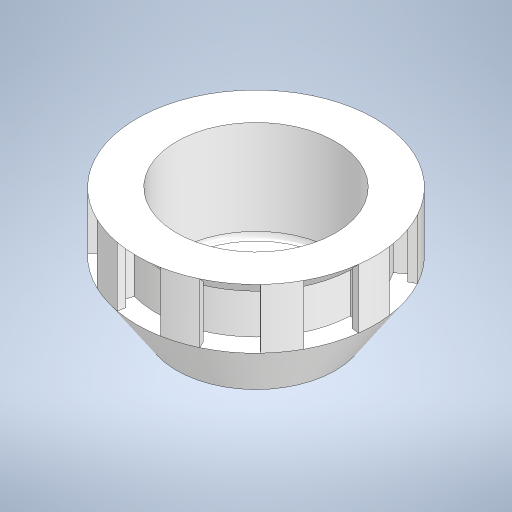
# Autodesk Inventor part: Tire Hub
Saved by Autodesk Inventor 2023.2 (Build 272271000, 271)
## iProperties
Created: 2023-02-06
Part Number: Tire Hub
Material: Nylon 6/6
Document SubType Name: Modeling
Designer: Nathan Cai
Density: 1.13 g/cm^3
Appearance: Smooth - White
Mass: 9.60807 g
Surface Area: 58.4208 cm^2
Volume: 8.50272 cm^3
Author: Nathan Cai
Autodesk Inventor part; units mm, degrees
ref_plane "YZ Plane" through (0, 0, 0) normal (1, 0, 0) x (0, 1, 0)
ref_plane "XZ Plane" through (0, 0, 0) normal (0, 1, 0) x (-1, 0, 0)
ref_plane "XY Plane" through (0, 0, 0) normal (0, 0, 1) x (1, 0, 0)
sketch "Sketch1" plane through (0, 0, 0) normal (0, 0, 1) x (1, 0, 0)
  line L0 (0, 19.05) -> (15.875, 19.05)
  line L1 (0, 9.525) -> (15.875, 9.525)
  line L2 (15.875, 19.05) -> (15.875, 9.525)
  line L3 (0, 0) -> (0, 19.05)
  line L4 (0, 19.05) -> (12.7, 19.05)
  line L5 (0, 0) -> (12.7, 0)
  line L6 (12.7, 0) -> (12.7, 19.05)
  line L7 (12.7, 19.05) -> (0, 19.05)
  line L8 (0, 19.05) -> (0, 0)
  line L9 (12.7, 3.175) -> (0, 3.175)
  line L10 (14.2875, 19.05) -> (14.2875, 9.525)
  line L11 (12.7, 0) -> (15.875, 0)
  line L12 (15.875, 0) -> (15.875, 9.525)
  line L13 (15.875, 9.525) -> (12.7, 9.525)
  line L14 (12.7, 9.525) -> (12.7, 0)
  line L15 (15.875, 0) -> (19.05, 9.525)
  line L16 (19.05, 9.525) -> (15.875, 9.525)
  line L17 (19.05, 9.525) -> (12.7, 0)
  point P0 (0, 3.175)
  dimension "d2" = 15.875
  dimension "d3" = 9.525
  dimension "d5" = 12.7
  dimension "d6" = 19.05
  dimension "d7" = 3.175
  dimension "d8" = 1.5875
  dimension "d21" = 19.05
  constraints: 36 end point, 6 horizontal, 4 parallel, 4 perpendicular, 4 point on line, 2 vertical
  measures "d2" distance of L0.start L0.end
  measures "d3" distance between parallel lines of L1 L0
  measures "d5" distance of L7.end L4.end
  measures "d6" distance between parallel lines of L5 L0
  measures "d7" distance between parallel lines of L5 L9
  measures "d8" distance between parallel lines of L2 L10
  measures "d21" distance from line of L3 L15.end
revolve "Revolution1" add sketch "Sketch1" angle 360 about axis through (0, 0, 0) along (0, 1, 0) contours L0 L10 L1 L6 | L0 L2 L1 L10 | L1 L12 L17 L6 | L9 L6 L5 L3 | L16 L17 L12
sketch "Sketch2" plane through (0, 0, 0) normal (0, -1, 0) x (1, 0, 0)
  circle A0 centre (0, 0) radius 3.302
  line L0 (0, 0) -> (0, -7.9375) construction
  circle A1 centre (0, -7.9375) radius 1.7526
  circle A2 centre (0, 7.9375) radius 1.7526
  point P0 (0, 0)
  dimension "d10" = 6.604
  dimension "d11" = 7.9375
  dimension "d12" = 3.5052
  dimension "d15" = 360
  constraints: 3 centre point, 2 coincident, 2 end point, 1 vertical, 5 other
  measures "d10" diameter of A0
  measures "d11" distance of L0.start L0.end
  measures "d12" diameter of A1
extrude "Extrusion1" cut sketch "Sketch2" against normal blind 25.4
fillet "Fillet1" radius 0.7937 1 edges at (-12.7, 3.175, 0)
chamfer "Chamfer1" distance 1.7272 angle 59 2 edges at (-1.7526, 0, 7.9375) (-1.7526, 0, -7.9375) measured on face at (-2.2526, 0, -7.9375) measured on face at (-2.2526, 0, 7.9375)
sketch "Sketch5" plane through (0, 19.05, 0) normal (0, 1, 0) x (1, 0, 0)
  circle A0 centre (0, 0) radius 19.05
  circle A1 centre (0, 0) radius 15.875
  dimension "d41" = 38.1
  constraints: 2 centre point, 1 coincident, 2 other
  measures "d41" diameter of A0
extrude "Extrusion3" add sketch "Sketch5" against normal blind 3.175
chamfer "Chamfer3" distance 3.175 angle 45 1 edges at (-19.05, 15.875, 0)
sketch "Sketch3" plane through (0, 9.525, 0) normal (0, 1, 0) x (1, 0, 0)
  circle A0 centre (0, 0) radius 19.05
  circle A1 centre (0, 0) radius 15.875
  circle A2 centre (0, 0) radius 17.8594
  line L0 (0, 0) -> (-19.0335, 0)
  line L1 (-19.0335, 0) -> (-19.0335, 0.7937) construction
  line L2 (-19.0335, 0.7937) -> (0, 0.7937)
  line L3 (0, 0.7937) -> (0, 0)
  line L4 (-19.0335, -0.7937) -> (0, -0.7937)
  circle A3 centre (0, 0) radius 19.05 projected
  line L5 (-17.7066, 2.3311) -> (-18.887, 2.4865)
  line L6 (-17.7066, -2.3311) -> (-18.887, -2.4865)
  line L7 (-15.8649, -10.5454) -> (-0.4666, 0.6422)
  line L8 (-14.9318, -11.8297) -> (0.4666, -0.6422)
  line L9 (-12.9547, -12.2936) -> (-13.8184, -13.1132)
  line L10 (-15.6951, -8.5218) -> (-16.7415, -9.0899)
  line L11 (-6.6366, -17.8566) -> (-0.7549, 0.2453)
  line L12 (-5.1268, -18.3472) -> (0.7549, -0.2453)
  line L13 (-3.2546, -17.5603) -> (-3.4716, -18.731)
  line L14 (-7.6887, -16.1196) -> (-8.2012, -17.1942)
  line L15 (5.1268, -18.3472) -> (-0.7549, -0.2453)
  line L16 (6.6366, -17.8566) -> (0.7549, 0.2453)
  line L17 (7.6887, -16.1196) -> (8.2012, -17.1942)
  line L18 (3.2546, -17.5603) -> (3.4716, -18.731)
  line L19 (14.9318, -11.8297) -> (-0.4666, -0.6422)
  line L20 (15.8649, -10.5454) -> (0.4666, 0.6422)
  line L21 (15.6951, -8.5218) -> (16.7415, -9.0899)
  line L22 (12.9547, -12.2936) -> (13.8184, -13.1132)
  line L23 (19.0335, -0.7938) -> (0, -0.7937)
  line L24 (19.0335, 0.7937) -> (0, 0.7937)
  line L25 (17.7066, 2.3311) -> (18.887, 2.4865)
  line L26 (17.7066, -2.3311) -> (18.887, -2.4865)
  line L27 (15.8649, 10.5454) -> (0.4666, -0.6422)
  line L28 (14.9318, 11.8297) -> (-0.4666, 0.6422)
  line L29 (12.9547, 12.2936) -> (13.8184, 13.1132)
  line L30 (15.6951, 8.5218) -> (16.7415, 9.0899)
  line L31 (6.6366, 17.8566) -> (0.7549, -0.2453)
  line L32 (5.1268, 18.3472) -> (-0.7549, 0.2453)
  line L33 (3.2546, 17.5603) -> (3.4716, 18.731)
  line L34 (7.6887, 16.1196) -> (8.2012, 17.1942)
  line L35 (-5.1268, 18.3472) -> (0.7549, 0.2453)
  line L36 (-6.6366, 17.8566) -> (-0.7549, -0.2453)
  line L37 (-7.6887, 16.1196) -> (-8.2012, 17.1942)
  line L38 (-3.2546, 17.5603) -> (-3.4716, 18.731)
  line L39 (-14.9318, 11.8297) -> (0.4666, 0.6422)
  line L40 (-15.8649, 10.5454) -> (-0.4666, -0.6422)
  line L41 (-15.6951, 8.5218) -> (-16.7415, 9.0899)
  line L42 (-12.9547, 12.2936) -> (-13.8184, 13.1132)
  point P0 (-13.9677, -11.1293)
  point P1 (-12.3605, -9.9616)
  point P2 (-13.2936, -8.6773)
  point P3 (-14.9008, -9.8449)
  point P4 (-4.7585, -17.2138)
  point P5 (-4.1446, -15.3244)
  point P6 (-5.6544, -14.8339)
  point P7 (-6.2683, -16.7232)
  point P8 (6.2683, -16.7232)
  point P9 (5.6544, -14.8339)
  point P10 (4.1446, -15.3244)
  point P11 (4.7585, -17.2138)
  point P12 (14.9008, -9.8449)
  point P13 (13.2936, -8.6773)
  point P14 (12.3605, -9.9616)
  point P15 (13.9677, -11.1293)
  point P16 (17.8417, 0.7937)
  point P17 (15.8551, 0.7937)
  point P18 (15.8551, -0.7938)
  point P19 (17.8417, -0.7938)
  point P20 (13.9677, 11.1293)
  point P21 (12.3605, 9.9616)
  point P22 (13.2936, 8.6773)
  point P23 (14.9008, 9.8449)
  point P24 (4.7585, 17.2138)
  point P25 (4.1446, 15.3244)
  point P26 (5.6544, 14.8339)
  point P27 (6.2683, 16.7232)
  point P28 (-6.2683, 16.7232)
  point P29 (-5.6544, 14.8339)
  point P30 (-4.1446, 15.3244)
  point P31 (-4.7585, 17.2138)
  point P32 (-14.9008, 9.8449)
  point P33 (-13.2936, 8.6773)
  point P34 (-12.3605, 9.9616)
  point P35 (-13.9677, 11.1293)
  point P36 (-17.8417, -0.7938)
  point P37 (-15.8551, -0.7938)
  point P38 (-15.8551, 0.7937)
  point P39 (-17.8417, 0.7937)
  dimension "d25" = 38.1
  dimension "d27" = 1.1906
  dimension "d26" = 31.75
  dimension "d28" = 0.7937
  dimension "d30" = 7.5
  dimension "d33" = 360
  constraints: 86 end point, 10 point on line, 4 symmetric about line, 3 coincident, 2 parallel, 1 centre point, 1 horizontal, 1 perpendicular, 1 point on circle, 137 other
  measures "d26" diameter of A1
  measures "d28" distance of L0.end L1.end
  measures "d30" angle of L0 L5
extrude "Extrusion2" add sketch "Sketch3" along normal up to surface (9.525 mm away) contours A0 L23 A2 L24 | L24 A2 L25 A0 | A0 L26 A2 L23 | A2 L23 A1 L24 | L30 A2 L27 A0 | A0 L20 A2 L21 | L27 A2 L28 A0 | A1 L28 A2 L27 | A0 L19 A2 L20 | L20 A2 L19 A1 | L28 A2 L29 A0 | A0 L22 A2 L19 | A1 L32 A2 L31 | L16 A2 L15 A1 | L34 A2 L31 A0 | A2 L32 A0 L31 | A0 L16 A2 L17 | L16 A0 L15 A2 | A1 L36 A2 L35 | A2 L33 A0 L32 | L12 A2 L11 A1 | L15 A0 L18 A2 | L35 A0 L38 A2 | A2 L36 A0 L35 | L12 A0 L11 A2 | A2 L13 A0 L12 | A1 L40 A2 L39 | A2 L37 A0 L36 | L8 A2 L7 A1 | L11 A0 L14 A2 | L39 A0 L42 A2 | A2 L40 A0 L39 | L8 A0 L7 A2 | A2 L9 A0 L8 | A1 L0 A2 L2 | A2 L41 A0 L40 | A1 L4 A2 L0 | L7 A0 L10 A2 | L2 A0 L5 A2 | A2 L4 A0 L2 | A2 L6 A0 L4
body "Solid1"
